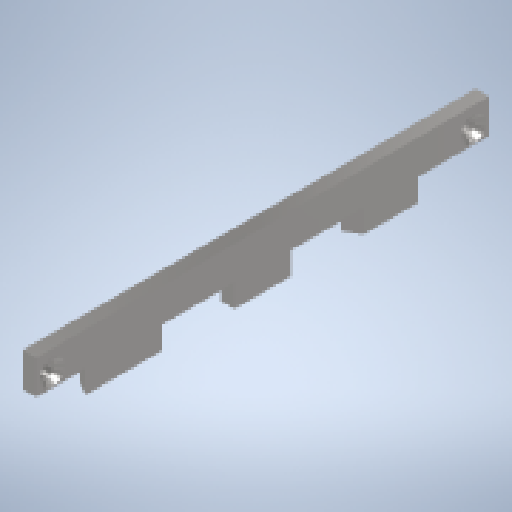
# Autodesk Inventor part: przod
Saved by Autodesk Inventor 2023.5 (Build 275446000, 446)
## iProperties
Created: 2025-01-11
Part Number: przod
Material: Stal, odlew
Document SubType Name: Modeling
Designer: kamil
Density: 7.85 g/cm^3
Appearance: Częściowo polerowany
Author: kamil
Autodesk Inventor part; units mm, degrees
ref_plane "YZ Plane" through (0, 0, 0) normal (1, 0, 0) x (0, 1, 0)
ref_plane "XZ Plane" through (0, 0, 0) normal (0, 1, 0) x (-1, 0, 0)
ref_plane "XY Plane" through (0, 0, 0) normal (0, 0, 1) x (1, 0, 0)
sketch "Szkic1" plane through (0, 0, 0) normal (1, 0, 0) x (0, 1, 0)
  line L0 (0, 0) -> (10.93, 0)
  line L1 (10.93, 0) -> (10.93, -100)
  line L2 (10.93, -100) -> (0, -100)
  line L3 (0, -100) -> (0, 0)
  dimension "d0" = 10.93
  dimension "d1" = 100
  constraints: 8 end point, 2 parallel, 1 horizontal, 1 perpendicular
  measures "d0" distance of L1.end L2.end
  measures "d1" distance of L0.end L1.end
extrude "Wyciągnięcie proste1" add sketch "Szkic1" along normal blind 3
sketch "Szkic2" plane through (0, 0, -100) normal (0, -1, 0) x (1, 0, 0)
  line L0 (-5, 84) -> (-8.1113, 87.1113) projected
  line L1 (-5, 84) -> (-4.2222, 84.7778) projected
  line L2 (-8.1113, 87.1113) -> (-7.3335, 87.8891) projected
  line L3 (-2, 60) -> (-3.1388, 64.2501) projected
  line L4 (-2, 60) -> (-0.9375, 60.2847) projected
  line L5 (-3.1388, 64.2501) -> (-2.0763, 64.5348) projected
  line L6 (-3.1388, 35.7499) -> (-2, 40) projected
  line L7 (-3.1388, 35.7499) -> (-2.0763, 35.4652) projected
  line L8 (-2, 40) -> (-0.9375, 39.7153) projected
  line L9 (-8.1113, 12.8887) -> (-5, 16) projected
  line L10 (-8.1113, 12.8887) -> (-7.3335, 12.1109) projected
  line L11 (-5, 16) -> (-4.2222, 15.2222) projected
  line L12 (-30.0489, 4.1) -> (-25.6489, 4.1) projected
  line L13 (-30.0489, 4.1) -> (-30.0489, 3) projected
  line L14 (-25.6489, 4.1) -> (-25.6489, 3) projected
  line L15 (-1.7913, 81.5519) -> (-5, 78.3431)
  line L16 (-5, 78.3431) -> (-13.7681, 87.1113)
  line L17 (-13.7681, 87.1113) -> (-10.5594, 90.32)
  line L18 (-10.5594, 90.32) -> (185.0217, 443.1577)
  arc A0 (351.0464, 277.133) -> (185.0217, 443.1577) centre (-11.203, 80.9083) ccw
  line L19 (351.0464, 277.133) -> (-1.7913, 81.5519)
  arc A1 (402.9118, 49.2349) -> (342.1425, 276.0288) centre (-8.9178, 60.424) ccw
  line L20 (402.9118, 49.2349) -> (-0.4452, 56.2755)
  line L21 (-0.4452, 56.2755) -> (-4.8284, 55.101)
  line L22 (-4.8284, 55.101) -> (-8.0378, 67.0785)
  line L23 (-8.0378, 67.0785) -> (-3.6546, 68.253)
  line L24 (-3.6546, 68.253) -> (342.1425, 276.0288)
  arc A2 (342.1425, -176.0288) -> (402.9118, 50.7651) centre (-8.9178, 39.576) ccw
  line L25 (342.1425, -176.0288) -> (-3.6546, 31.747)
  line L26 (-3.6546, 31.747) -> (-8.0378, 32.9215)
  line L27 (-8.0378, 32.9215) -> (-4.8284, 44.899)
  line L28 (-4.8284, 44.899) -> (-0.4452, 43.7245)
  line L29 (-0.4452, 43.7245) -> (402.9118, 50.7651)
  arc A3 (185.0217, -343.1577) -> (351.0464, -177.133) centre (-11.203, 19.0917) ccw
  line L30 (185.0217, -343.1577) -> (-10.5594, 9.68)
  line L31 (-10.5594, 9.68) -> (-13.7681, 12.8887)
  line L32 (-13.7681, 12.8887) -> (-5, 21.6569)
  line L33 (-5, 21.6569) -> (-1.7913, 18.4481)
  line L34 (-1.7913, 18.4481) -> (351.0464, -177.133)
  line L35 (-25.6489, 3) -> (-30.0489, 3) projected
  line L36 (-0.9375, 39.7153) -> (-2.0763, 35.4652) projected
  line L37 (-7.3335, 87.8891) -> (-4.2222, 84.7778) projected
  line L38 (-4.2222, 15.2222) -> (-7.3335, 12.1109) projected
  line L39 (-2.0763, 64.5348) -> (-0.9375, 60.2847) projected
  point P0 (0, 100)
  point P1 (259.8393, 226.5761)
  point P2 (359.0779, 50)
  point P3 (259.8393, -126.5761)
  point P4 (343.886, -173.1639)
  point P5 (402.9318, 50)
  point P6 (343.886, 273.1639)
  constraints: 40 end point, 8 point on circle, 4 centre point, 8 other
extrude "Wyciągnięcie proste2" cut sketch "Szkic2" against normal blind 5 contours L0 L2 L37 L1 | L3 L5 L39 L4 | L6 L8 L36 L7 | L9 L11 L38 L10 | L15 L16 L17 L18 A0 L19 A1 L24 | L24 A1 L19 | L19 A1 A2 L29 L20 L21 L22 L23 L24 | A2 L34 L25 L26 L27 L28 L29 L20 A1 | A1 L20 L29 A2 | L34 A3 L30 L31 L32 L33 L25 A2 | A2 L25 L34
sketch "Szkic3" plane through (3, 0, 0) normal (1, 0, 0) x (0, 0, -1)
  circle A0 centre (3.5, 7.9652) radius 2 projected
  circle A1 centre (96.5, 7.9652) radius 2 projected
  point P0 (0, 0)
hole "Otwór1" at (3, 7.9652, -3.5) at (3, 7.9652, -96.5) direction (-1, 0, 0) diameter 3.2 depth 5 tip angle 118 countersink diameter 5.5 countersink angle 90
sketch "Szkic4" plane through (0, 5, -100) normal (0, -1, 0) x (1, 0, 0)
  line L0 (3, 100) -> (3, 84.2077) projected
  line L1 (0, 100) -> (3, 100) projected
  line L2 (0, 82.5448) -> (0, 100) projected
  line L3 (3, 84.2077) -> (0, 82.5448) projected
extrude "Wyciągnięcie proste3" add sketch "Szkic4" along normal up to surface (5 mm away)
sketch "Szkic5" plane through (0, 0, 0) normal (0, -1, 0) x (1, 0, 0)
  line L0 (4.8201, -9.9008) -> (54.794, 17.8002) projected
  line L1 (4.8201, -9.9008) -> (-21.7144, -24.6091)
  line L2 (-21.7144, -24.6091) -> (-5.6558, 14.396)
  line L3 (-5.6558, 14.396) -> (27.8601, 2.8705)
  line L4 (3, 0) -> (3, -27.7486) projected
  line L5 (0, 0) -> (0, -29.5511) projected
  line L6 (3, 0) -> (0, 0) projected
  point P0 (0, -12.5726)
  point P1 (3, -10.9097)
  constraints: 6 end point, 1 collinear, 1 point on line
extrude "Wyciągnięcie proste4" cut sketch "Szkic5" against normal up to surface (5 mm away) contours L1 L5 L6 L4
sketch "Szkic6" plane through (0, 10.93, 0) normal (0, 1, 0) x (1, 0, 0)
  line L0 (0, 100) -> (0, 0) projected
  line L1 (0, 0) -> (3, 0) projected
  line L2 (3, 100) -> (3, 0) projected
  line L3 (0, 100) -> (3, 100) projected
  point P0 (0, 0)
ref_plane "Płaszczyzna konstrukcyjna1" through (-44.8489, 12.5303, -7) normal (0, 1, 0) x (0, 0, 1)
extrude "Wyciągnięcie proste5" add sketch "Szkic6" along normal up to surface (1.6003 mm away)
